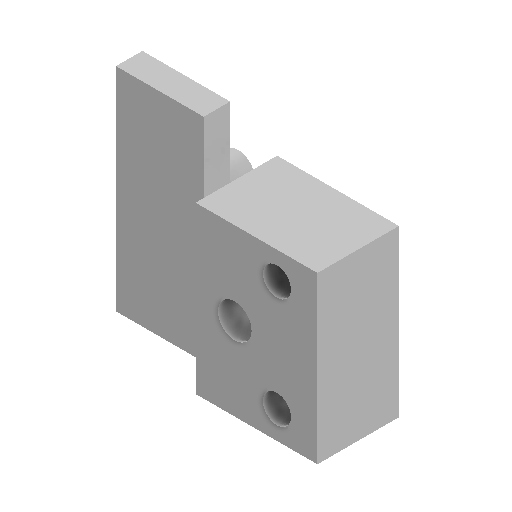
# Autodesk Inventor part: 00_Linear_Stepper_90mm_slide
Saved by Autodesk Inventor 2022 (Build 260153000, 153)
## iProperties
Created: 2021-12-21
Part Number: 00_Linear_Stepper_90mm_slide
Material: Generisch
Document SubType Name: Modeling
Designer: diederichbenedict
Density: 1 g/cm^3
Appearance: Vorgabe
Author: diederichbenedict
Autodesk Inventor part; units mm, degrees
ref_plane "YZ Plane" through (0, 0, 0) normal (1, 0, 0) x (0, 1, 0)
ref_plane "XZ Plane" through (0, 0, 0) normal (0, 1, 0) x (-1, 0, 0)
ref_plane "XY Plane" through (0, 0, 0) normal (0, 0, 1) x (1, 0, 0)
sketch "Skizze1" plane through (0, 0, 0) normal (0, 0, 1) x (1, 0, 0)
  circle A0 centre (-2.545, 0) radius 7.475 projected
  circle A1 centre (-2.545, 0) radius 1.5 projected
  circle A2 centre (1.205, -4.91) radius 1.25 projected
  circle A3 centre (1.205, 4.91) radius 1.25 projected
  line L0 (-6.025, -7.365) -> (4.805, -7.365)
  line L1 (4.805, -7.365) -> (4.805, 7.365)
  line L2 (4.805, 7.365) -> (-6.025, 7.365)
  line L3 (-6.025, 7.365) -> (-6.025, -7.365)
  line L4 (-6.025, -7.365) -> (4.805, 7.365) construction
  line L5 (4.805, -7.365) -> (-6.025, 7.365) construction
  line L6 (-10.205, -1.8) -> (-6.025, -1.8)
  line L7 (-6.025, -1.8) -> (-6.025, 1.8)
  line L8 (-6.025, 1.8) -> (-10.205, 1.8)
  line L9 (-10.205, 1.8) -> (-10.205, -1.8)
  line L10 (-10.205, -1.8) -> (-6.025, 1.8) construction
  line L11 (-6.025, -1.8) -> (-10.205, 1.8) construction
  line L12 (-18.005, -9.44) -> (-10.205, -9.44)
  line L13 (-10.205, -9.44) -> (-10.205, 9.44)
  line L14 (-10.205, 9.44) -> (-18.005, 9.44)
  line L15 (-18.005, 9.44) -> (-18.005, -9.44)
  line L16 (-18.005, -9.44) -> (-10.205, 9.44) construction
  line L17 (-10.205, -9.44) -> (-18.005, 9.44) construction
  point P0 (0, 0)
  point P1 (-0.61, 0)
  point P2 (-8.115, 0)
  point P3 (-6.025, 0)
  point P4 (-14.105, 0)
  point P5 (-10.205, 0)
  dimension "d1" = 3.6
  dimension "d2" = 14.73
  dimension "d3" = 10.83
  dimension "d4" = 4.18
  dimension "d5" = 3.6
  dimension "d6" = 18.88
  dimension "d7" = 7.8
  constraints: 36 end point, 10 midpoint, 6 parallel, 3 horizontal, 3 perpendicular
  measures "d1" distance from line of L1 A3.centre
  measures "d2" distance between parallel lines of L0 L2
  measures "d3" distance between parallel lines of L3 L1
  measures "d4" distance of L8.end L7.end
  measures "d5" distance of L7.end L6.end
  measures "d6" distance between parallel lines of L12 L14
  measures "d7" distance between parallel lines of L15 L13
extrude "Extrusion1" add sketch "Skizze1" along normal blind 2.35 contours L1 A0 L0 L3 L2 | A0 L2 L1 | L1 L0 A0 | A0 L3 L2 | L0 L3 A0 | L8 L3 L6 A0 | A0 L6 L9 L8 | L9 L13 L12 L15 L14
sketch "Skizze2" plane through (0, 0, 2.35) normal (0, 0, 1) x (1, 0, 0)
  line L0 (-10.205, -9.44) -> (-10.205, -1.8) projected
  line L1 (-10.205, -1.8) -> (-6.025, -1.8) projected
  line L2 (-6.025, -1.8) -> (-6.025, -7.365) projected
  line L3 (-6.025, -7.365) -> (4.805, -7.365) projected
  line L4 (4.805, -7.365) -> (4.805, 7.365) projected
  line L5 (4.805, 7.365) -> (-6.025, 7.365) projected
  line L6 (-6.025, 7.365) -> (-6.025, 1.8) projected
  line L7 (-6.025, 1.8) -> (-10.205, 1.8) projected
  line L8 (-10.205, 1.8) -> (-10.205, 9.44) projected
  line L9 (-10.205, 9.44) -> (-18.005, 9.44) projected
  line L10 (-18.005, 9.44) -> (-18.005, -9.44) projected
  line L11 (-18.005, -9.44) -> (-10.205, -9.44) projected
  circle A0 centre (1.205, 4.91) radius 1.25 projected
  circle A1 centre (1.205, -4.91) radius 1.25 projected
  circle A2 centre (-2.545, 0) radius 1.5 projected
  line L12 (-6.025, 1.8) -> (-10.205, 1.8) projected
  line L13 (-6.025, 1.8) -> (-6.025, -1.8)
  point P0 (0, 0)
  constraints: 2 end point, 1 perpendicular
extrude "Extrusion2" add sketch "Skizze2" along normal blind 4.9 contours L13 L6 L5 L4 L3 L2
sketch "Skizze3" plane through (0, 0, 0) normal (0, 0, -1) x (-1, 0, 0)
  line L0 (10.205, -9.44) -> (10.205, -1.8) projected
  line L1 (18.005, -9.44) -> (10.205, -9.44) projected
  line L2 (18.005, 9.44) -> (18.005, -9.44) projected
  line L3 (10.205, 9.44) -> (18.005, 9.44) projected
  line L4 (10.205, 1.8) -> (10.205, 9.44) projected
  line L5 (6.025, 1.8) -> (10.205, 1.8) projected
  line L6 (6.025, 7.365) -> (6.025, 1.8) projected
  line L7 (-4.805, 7.365) -> (6.025, 7.365) projected
  line L8 (-4.805, -7.365) -> (-4.805, 7.365) projected
  line L9 (6.025, -7.365) -> (-4.805, -7.365) projected
  line L10 (6.025, -1.8) -> (6.025, -7.365) projected
  line L11 (10.205, -1.8) -> (6.025, -1.8) projected
  circle A0 centre (-1.205, 4.91) radius 1.25 projected
  circle A1 centre (-1.205, -4.91) radius 1.25 projected
  circle A2 centre (2.545, 0) radius 1.5 projected
  circle A3 centre (14.105, 0) radius 1.435
  point P0 (0, 0)
  dimension "d12" = 2.87
  constraints: 1 centre point
  measures "d12" diameter of A3
extrude "Extrusion3" add sketch "Skizze3" along normal blind 4.64 contours A3
